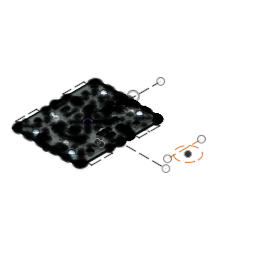
麦轮小车底盘上板-可编辑 (Autodesk Fusion 360 design; units mm, degrees)
Autodesk Fusion 360 part; units mm, degrees
(part 1 of 2)
sketch "草图1" plane through (0, 0, 0) normal (0, 0, 1) x (1, 0, 0)
  circle A0 centre (53, 101) radius 2.1
  line L0 (45.5, 106) -> (86.5, 106) construction
  line L1 (86.5, 106) -> (86.5, 66) construction
  line L2 (86.5, 66) -> (45.5, 66) construction
  line L3 (45.5, 66) -> (45.5, 106) construction
  circle A1 centre (78, 101) radius 2.1
  circle A2 centre (53, 71) radius 2.1
  circle A3 centre (78, 71) radius 2.1
  line L4 (83.5, 106) -> (83.5, 66) construction
  circle A4 centre (277.8426, 86) radius 37.5 construction
  line L5 (86.5, 86) -> (45.5, 86) construction
  line L6 (255.8426, 157.1035) -> (255.8426, 33.728) construction
  line L7 (0, 0) -> (284.0564, 0) construction
  line L8 (0, 0) -> (0, 265.0446) construction
  line L9 (122, 150) -> (-122, 150) construction
  line L10 (-122, 150) -> (-122, -150)
  line L11 (-122, -150) -> (122, -150) construction
  line L12 (122, -150) -> (122, 150)
  line L13 (122, 150) -> (-122, -150) construction
  line L14 (-122, 150) -> (122, -150) construction
  line L15 (13.5, 100) -> (45.5, 100) construction
  line L16 (45.5, 100) -> (45.5, 72) construction
  line L17 (45.5, 72) -> (13.5, 72) construction
  line L18 (13.5, 72) -> (13.5, 100) construction
  line L19 (86.5, 100) -> (106, 100) construction
  line L20 (106, 100) -> (106, 72) construction
  line L21 (106, 72) -> (86.5, 72) construction
  line L22 (86.5, 72) -> (86.5, 100) construction
  line L23 (106, 123.5) -> (138, 123.5) construction
  line L24 (138, 123.5) -> (138, 48.5) construction
  line L25 (138, 48.5) -> (106, 48.5) construction
  line L26 (106, 48.5) -> (106, 123.5) construction
  line L27 (86.5, 86) -> (138, 86) construction
  circle A5 centre (40.5, 61) radius 5 construction
  line L28 (-106, 123.5) -> (-138, 123.5) construction
  line L29 (-106, 48.5) -> (-106, 123.5) construction
  line L30 (-138, 48.5) -> (-106, 48.5) construction
  line L31 (-138, 123.5) -> (-138, 48.5) construction
  line L32 (-138, -123.5) -> (-138, -48.5) construction
  line L33 (-106, -123.5) -> (-138, -123.5) construction
  line L34 (-106, -48.5) -> (-106, -123.5) construction
  line L35 (-138, -48.5) -> (-106, -48.5) construction
  line L36 (106, -48.5) -> (106, -123.5) construction
  line L37 (106, -123.5) -> (138, -123.5) construction
  line L38 (138, -123.5) -> (138, -48.5) construction
  line L39 (138, -48.5) -> (106, -48.5) construction
  line L40 (117, 126.5) -> (99, 126.5) construction
  line L41 (96, 123.5) -> (96, 86) construction
  arc A6 (99, 126.5) -> (96, 123.5) centre (99, 123.5) ccw construction
  line L42 (96, 48.5) -> (96, 86) construction
  arc A7 (96, 48.5) -> (99, 45.5) centre (99, 48.5) ccw construction
  line L43 (117, 45.5) -> (99, 45.5) construction
  line L44 (122, 131.5) -> (122, 140)
  line L45 (112, 150) -> (0, 150)
  line L46 (122, 40.5) -> (122, 0)
  arc A8 (117, 126.5) -> (122, 131.5) centre (117, 131.5) ccw construction
  arc A9 (122, 40.5) -> (117, 45.5) centre (117, 40.5) ccw construction
  arc A10 (122, 140) -> (112, 150) centre (112, 140) ccw
  line L47 (-117, 45.5) -> (-99, 45.5) construction
  arc A11 (-99, 45.5) -> (-96, 48.5) centre (-99, 48.5) ccw construction
  line L48 (-122, 40.5) -> (-122, 0)
  arc A12 (-117, 45.5) -> (-122, 40.5) centre (-117, 40.5) ccw construction
  line L49 (-96, 48.5) -> (-96, 86) construction
  line L50 (-96, 123.5) -> (-96, 86) construction
  arc A13 (-96, 123.5) -> (-99, 126.5) centre (-99, 123.5) ccw construction
  line L51 (-117, 126.5) -> (-99, 126.5) construction
  arc A14 (-122, 131.5) -> (-117, 126.5) centre (-117, 131.5) ccw construction
  line L52 (-122, 131.5) -> (-122, 140)
  arc A15 (-112, 150) -> (-122, 140) centre (-112, 140) ccw
  line L53 (-112, 150) -> (0, 150)
  line L54 (-96, -123.5) -> (-96, -86) construction
  line L55 (-96, -48.5) -> (-96, -86) construction
  line L56 (-117, -45.5) -> (-99, -45.5) construction
  arc A16 (-96, -48.5) -> (-99, -45.5) centre (-99, -48.5) ccw construction
  arc A17 (-122, -40.5) -> (-117, -45.5) centre (-117, -40.5) ccw construction
  line L57 (-122, -40.5) -> (-122, 0)
  arc A18 (-99, -126.5) -> (-96, -123.5) centre (-99, -123.5) ccw construction
  line L58 (-117, -126.5) -> (-99, -126.5) construction
  arc A19 (-117, -126.5) -> (-122, -131.5) centre (-117, -131.5) ccw construction
  line L59 (-122, -131.5) -> (-122, -140)
  arc A20 (-122, -140) -> (-112, -150) centre (-112, -140) ccw
  line L60 (-112, -150) -> (0, -150)
  line L61 (112, -150) -> (0, -150)
  arc A21 (112, -150) -> (122, -140) centre (112, -140) ccw
  line L62 (122, -131.5) -> (122, -140)
  arc A22 (122, -131.5) -> (117, -126.5) centre (117, -131.5) ccw construction
  line L63 (117, -126.5) -> (99, -126.5) construction
  arc A23 (96, -123.5) -> (99, -126.5) centre (99, -123.5) ccw construction
  line L64 (96, -123.5) -> (96, -86) construction
  line L65 (96, -48.5) -> (96, -86) construction
  arc A24 (99, -45.5) -> (96, -48.5) centre (99, -48.5) ccw construction
  line L66 (117, -45.5) -> (99, -45.5) construction
  arc A25 (117, -45.5) -> (122, -40.5) centre (117, -40.5) ccw construction
  line L67 (122, -40.5) -> (122, 0)
  circle A26 centre (-40.5, 61) radius 5 construction
  circle A27 centre (-78, 71) radius 2.1
  circle A28 centre (-53, 71) radius 2.1
  circle A29 centre (-53, 101) radius 2.1
  circle A30 centre (-78, 101) radius 2.1
  circle A31 centre (40.5, -61) radius 5
  circle A32 centre (-40.5, -61) radius 5
  line L68 (-99, 45.5) -> (99, 45.5) construction
  line L69 (-96, 48.5) -> (-96, 45.5) construction
  line L70 (96, 48.5) -> (96, 45.5) construction
  line L71 (-93, 48.5) -> (93, 48.5) construction
  line L72 (-96, 86) -> (-96, 51.5) construction
  line L73 (96, 86) -> (96, 51.5) construction
  arc A33 (93, 48.5) -> (96, 51.5) centre (93, 51.5) ccw construction
  arc A34 (-96, 51.5) -> (-93, 48.5) centre (-93, 51.5) ccw construction
  line L74 (8, 91) -> (-8, 91) construction
  arc A35 (-8, 91) -> (-8, 81) centre (-8, 86) ccw construction
  line L75 (-8, 81) -> (8, 81) construction
  arc A36 (8, 81) -> (8, 91) centre (8, 86) ccw construction
  line L76 (8, 86) -> (-8, 86) construction
  line L77 (-8, -81) -> (8, -81)
  arc A37 (-8, -81) -> (-8, -91) centre (-8, -86) ccw
  line L78 (8, -91) -> (-8, -91)
  arc A38 (8, -91) -> (8, -81) centre (8, -86) ccw
  circle A39 centre (-78, -71) radius 2.1
  circle A40 centre (-78, -101) radius 2.1
  circle A41 centre (-53, -101) radius 2.1
  circle A42 centre (-53, -71) radius 2.1
  circle A43 centre (53, -101) radius 2.1
  circle A44 centre (78, -101) radius 2.1
  circle A45 centre (78, -71) radius 2.1
  circle A46 centre (53, -71) radius 2.1
  circle A47 centre (-112, 140) radius 2.1
  circle A48 centre (112, 140) radius 2.1
  circle A49 centre (-112, -140) radius 2.1
  circle A50 centre (112, -140) radius 2.1
  line L79 (92, 53) -> (87, 53) construction
  arc A51 (87, 53) -> (87, 50) centre (87, 51.5) ccw construction
  line L80 (87, 50) -> (92, 50) construction
  arc A52 (92, 50) -> (92, 53) centre (92, 51.5) ccw construction
  line L81 (92, 51.5) -> (87, 51.5) construction
  line L82 (92, 44) -> (87, 44) construction
  arc A53 (87, 44) -> (87, 41) centre (87, 42.5) ccw construction
  line L83 (87, 41) -> (92, 41) construction
  arc A54 (92, 41) -> (92, 44) centre (92, 42.5) ccw construction
  line L84 (92, 42.5) -> (87, 42.5) construction
  line L85 (-87, 50) -> (-92, 50) construction
  arc A55 (-87, 50) -> (-87, 53) centre (-87, 51.5) ccw construction
  line L86 (-92, 53) -> (-87, 53) construction
  arc A56 (-92, 53) -> (-92, 50) centre (-92, 51.5) ccw construction
  line L87 (-92, 44) -> (-87, 44) construction
  arc A57 (-87, 41) -> (-87, 44) centre (-87, 42.5) ccw construction
  line L88 (-87, 41) -> (-92, 41) construction
  arc A58 (-92, 44) -> (-92, 41) centre (-92, 42.5) ccw construction
  circle A59 centre (20.5, 39.5) radius 2.75 construction
  circle A60 centre (16, 54) radius 2.9 construction
  circle A61 centre (-16, 54) radius 2.9 construction
  circle A62 centre (-20.5, 39.5) radius 2.75 construction
  circle A63 centre (15.25, 15.25) radius 1.55
  circle A64 centre (22.5, 22.5) radius 1.55
  line L89 (0, 0) -> (46.5904, 46.5904) construction
  line L90 (0, 0) -> (50.6063, 0) construction
  circle A65 centre (-15.25, 15.25) radius 1.55
  circle A66 centre (-22.5, 22.5) radius 1.55
  circle A67 centre (22.5, -22.5) radius 1.55
  circle A68 centre (15.25, -15.25) radius 1.55
  circle A69 centre (-15.25, -15.25) radius 1.55
  circle A70 centre (-22.5, -22.5) radius 1.55
  circle A71 centre (0, 0) radius 5
  line L91 (116.45, 32.5) -> (116.45, 7.5)
  arc A72 (116.45, 7.5) -> (119.55, 7.5) centre (118, 7.5) ccw
  line L92 (119.55, 7.5) -> (119.55, 32.5)
  arc A73 (119.55, 32.5) -> (116.45, 32.5) centre (118, 32.5) ccw
  line L93 (118, 32.5) -> (118, 7.5) construction
  circle A74 centre (118, 0) radius 1.6
  circle A75 centre (118, 40) radius 1.6
  circle A76 centre (118, -40) radius 1.6
  line L94 (116.45, -32.5) -> (116.45, -7.5)
  arc A77 (116.45, -32.5) -> (119.55, -32.5) centre (118, -32.5) ccw
  line L95 (119.55, -7.5) -> (119.55, -32.5)
  arc A78 (119.55, -7.5) -> (116.45, -7.5) centre (118, -7.5) ccw
  circle A79 centre (-118, -40) radius 1.6
  arc A80 (-119.55, -32.5) -> (-116.45, -32.5) centre (-118, -32.5) ccw
  line L96 (-119.55, -7.5) -> (-119.55, -32.5)
  line L97 (-116.45, -32.5) -> (-116.45, -7.5)
  arc A81 (-116.45, -7.5) -> (-119.55, -7.5) centre (-118, -7.5) ccw
  circle A82 centre (-118, 0) radius 1.6
  arc A83 (-119.55, 7.5) -> (-116.45, 7.5) centre (-118, 7.5) ccw
  line L98 (-119.55, 7.5) -> (-119.55, 32.5)
  line L99 (-116.45, 32.5) -> (-116.45, 7.5)
  arc A84 (-116.45, 32.5) -> (-119.55, 32.5) centre (-118, 32.5) ccw
  circle A85 centre (-118, 40) radius 1.6
  line L100 (116.45, 141.5) -> (116.45, 131.5)
  arc A86 (116.45, 131.5) -> (119.55, 131.5) centre (118, 131.5) ccw
  line L101 (119.55, 131.5) -> (119.55, 141.5)
  arc A87 (119.55, 141.5) -> (116.45, 141.5) centre (118, 141.5) ccw
  line L102 (118, 141.5) -> (118, 131.5) construction
  line L103 (-119.55, 131.5) -> (-119.55, 141.5)
  line L104 (-116.45, 141.5) -> (-116.45, 131.5)
  arc A88 (-116.45, 141.5) -> (-119.55, 141.5) centre (-118, 141.5) ccw
  arc A89 (-119.55, 131.5) -> (-116.45, 131.5) centre (-118, 131.5) ccw
  line L105 (-15, 144.45) -> (15, 144.45)
  arc A90 (15, 144.45) -> (15, 147.55) centre (15, 146) ccw
  line L106 (15, 147.55) -> (-15, 147.55)
  arc A91 (-15, 147.55) -> (-15, 144.45) centre (-15, 146) ccw
  line L107 (-15, 146) -> (15, 146) construction
  circle A92 centre (22.5, 146) radius 1.6
  line L108 (30, 144.45) -> (60, 144.45)
  arc A93 (60, 144.45) -> (60, 147.55) centre (60, 146) ccw
  line L109 (60, 147.55) -> (30, 147.55)
  arc A94 (30, 147.55) -> (30, 144.45) centre (30, 146) ccw
  line L110 (30, 146) -> (60, 146) construction
  circle A95 centre (67.5, 146) radius 1.6
  line L111 (75, 144.45) -> (105, 144.45)
  arc A96 (105, 144.45) -> (105, 147.55) centre (105, 146) ccw
  line L112 (105, 147.55) -> (75, 147.55)
  arc A97 (75, 147.55) -> (75, 144.45) centre (75, 146) ccw
  line L113 (75, 146) -> (105, 146) construction
  circle A98 centre (112.5, 146) radius 1.6
  arc A99 (-30, 144.45) -> (-30, 147.55) centre (-30, 146) ccw
  line L114 (-60, 147.55) -> (-30, 147.55)
  arc A100 (-60, 147.55) -> (-60, 144.45) centre (-60, 146) ccw
  line L115 (-30, 144.45) -> (-60, 144.45)
  circle A101 centre (-67.5, 146) radius 1.6
  circle A102 centre (-22.5, 146) radius 1.6
  arc A103 (-75, 144.45) -> (-75, 147.55) centre (-75, 146) ccw
  line L116 (-105, 147.55) -> (-75, 147.55)
  line L117 (-75, 144.45) -> (-105, 144.45)
  arc A104 (-105, 147.55) -> (-105, 144.45) centre (-105, 146) ccw
  circle A105 centre (-112.5, 146) radius 1.6
  circle A106 centre (0, 135) radius 5
  circle A107 centre (40.5, 33) radius 5 construction
  circle A108 centre (45.5, 52.5) radius 1.5 construction
  line L118 (40.5, 61) -> (40.5, 33) construction
  circle A109 centre (35.5, 52.5) radius 1.5 construction
  circle A110 centre (35.5, 41.5) radius 1.5 construction
  circle A111 centre (45.5, 41.5) radius 1.5 construction
  circle A112 centre (-35.5, 52.5) radius 1.5 construction
  circle A113 centre (-45.5, 52.5) radius 1.5 construction
  circle A114 centre (-35.5, 41.5) radius 1.5 construction
  circle A115 centre (-45.5, 41.5) radius 1.5 construction
  circle A116 centre (-40.5, 33) radius 5 construction
  circle A117 centre (35.5, -52.5) radius 1.5
  circle A118 centre (45.5, -52.5) radius 1.5
  circle A119 centre (-35.5, -52.5) radius 1.5
  circle A120 centre (-45.5, -52.5) radius 1.5
  circle A121 centre (6, 76.5) radius 1.5
  circle A122 centre (-6, 76.5) radius 1.5
  circle A123 centre (0, 115) radius 25.5 construction
  circle A124 centre (0, 115) radius 19.8 construction
  line L119 (0, 115) -> (20.8597, 135.8596) construction
  line L120 (0, 115) -> (15.4307, 115) construction
  circle A125 centre (14.0007, 129.0007) radius 1.3
  circle A126 centre (-14.0007, 100.9993) radius 1.3
  circle A127 centre (0, 115) radius 29.5 construction
  circle A128 centre (20.8597, 135.8596) radius 1.6
  circle A129 centre (-20.8596, 135.8597) radius 1.6
  circle A130 centre (-20.8596, 94.1403) radius 1.6
  circle A131 centre (20.8597, 94.1403) radius 1.6
  circle A132 centre (-14.0007, 129.0007) radius 1.3
  circle A133 centre (14.0007, 100.9993) radius 1.3
  line L121 (-39.5, -73.5) -> (39.5, -73.5) construction
  line L122 (42.5, -76.5) -> (42.5, -126.5) construction
  line L123 (39.5, -129.5) -> (-39.5, -129.5) construction
  line L124 (-42.5, -126.5) -> (-42.5, -76.5) construction
  arc A134 (-39.5, -73.5) -> (-42.5, -76.5) centre (-39.5, -76.5) ccw construction
  arc A135 (42.5, -76.5) -> (39.5, -73.5) centre (39.5, -76.5) ccw construction
  arc A136 (39.5, -129.5) -> (42.5, -126.5) centre (39.5, -126.5) ccw construction
  arc A137 (-42.5, -126.5) -> (-39.5, -129.5) centre (-39.5, -126.5) ccw construction
  line L125 (-42.5, -101.5) -> (42.5, -101.5) construction
  circle A138 centre (-39, -77) radius 1.6
  circle A139 centre (-39, -126) radius 1.6
  circle A140 centre (19, -77) radius 1.6
  circle A141 centre (19, -126) radius 1.6
  line L126 (0, -73.5) -> (0, -129.5) construction
  circle A142 centre (-19, -77) radius 1.6
  circle A143 centre (39, -77) radius 1.6
  circle A144 centre (39, -126) radius 1.6
  circle A145 centre (-19, -126) radius 1.6
  line L127 (0, -101.5) -> (28.2843, -73.2157) construction
  line L128 (0, -101.5) -> (22.405, -101.5) construction
  circle A146 centre (24.5, -62.5) radius 1.6
  circle A147 centre (24.5, -82.5) radius 1.6
  circle A148 centre (24.5, -120.5) radius 1.6
  circle A149 centre (24.5, -140.5) radius 1.6
  circle A150 centre (-24.5, -140.5) radius 1.6
  circle A151 centre (-24.5, -120.5) radius 1.6
  circle A152 centre (-24.5, -82.5) radius 1.6
  circle A153 centre (-24.5, -62.5) radius 1.6
  circle A154 centre (-5, -61.5) radius 1.5
  circle A155 centre (5, -61.5) radius 1.5
  circle A156 centre (-5, -35) radius 1.5
  circle A157 centre (5, -35) radius 1.5
  circle A158 centre (5, 35) radius 1.5
  circle A159 centre (-5, 35) radius 1.5
  circle A160 centre (35, 5) radius 1.5
  circle A161 centre (35, -5) radius 1.5
  circle A162 centre (-35, 5) radius 1.5
  circle A163 centre (-35, -5) radius 1.5
  line L129 (-105, -147.55) -> (-75, -147.55)
  arc A164 (-105, -144.45) -> (-105, -147.55) centre (-105, -146) ccw
  circle A165 centre (-112.5, -146) radius 1.6
  line L130 (-75, -144.45) -> (-105, -144.45)
  arc A166 (-75, -147.55) -> (-75, -144.45) centre (-75, -146) ccw
  circle A167 centre (-67.5, -146) radius 1.6
  arc A168 (-60, -144.45) -> (-60, -147.55) centre (-60, -146) ccw
  line L131 (-60, -147.55) -> (-30, -147.55)
  line L132 (-30, -144.45) -> (-60, -144.45)
  arc A169 (-30, -147.55) -> (-30, -144.45) centre (-30, -146) ccw
  circle A170 centre (-22.5, -146) radius 1.6
  arc A171 (-15, -144.45) -> (-15, -147.55) centre (-15, -146) ccw
  line L133 (15, -147.55) -> (-15, -147.55)
  line L134 (-15, -144.45) -> (15, -144.45)
  arc A172 (15, -147.55) -> (15, -144.45) centre (15, -146) ccw
  circle A173 centre (22.5, -146) radius 1.6
  arc A174 (30, -144.45) -> (30, -147.55) centre (30, -146) ccw
  line L135 (60, -147.55) -> (30, -147.55)
  line L136 (30, -144.45) -> (60, -144.45)
  arc A175 (60, -147.55) -> (60, -144.45) centre (60, -146) ccw
  circle A176 centre (67.5, -146) radius 1.6
  arc A177 (75, -144.45) -> (75, -147.55) centre (75, -146) ccw
  line L137 (105, -147.55) -> (75, -147.55)
  line L138 (75, -144.45) -> (105, -144.45)
  arc A178 (105, -147.55) -> (105, -144.45) centre (105, -146) ccw
  circle A179 centre (112.5, -146) radius 1.6
  line L139 (116.45, -141.5) -> (116.45, -131.5)
  arc A180 (116.45, -141.5) -> (119.55, -141.5) centre (118, -141.5) ccw
  line L140 (119.55, -131.5) -> (119.55, -141.5)
  arc A181 (119.55, -131.5) -> (116.45, -131.5) centre (118, -131.5) ccw
  line L141 (-116.45, -141.5) -> (-116.45, -131.5)
  line L142 (-119.55, -131.5) -> (-119.55, -141.5)
  arc A182 (-119.55, -141.5) -> (-116.45, -141.5) centre (-118, -141.5) ccw
  arc A183 (-116.45, -131.5) -> (-119.55, -131.5) centre (-118, -131.5) ccw
  circle A184 centre (40, 140) radius 2.1
  circle A185 centre (-40, 140) radius 2.1
  circle A186 centre (-86, 58.5) radius 2.1
  circle A187 centre (86, 58.5) radius 2.1
  circle A188 centre (-112, 35.5) radius 2.1
  circle A189 centre (112, 35.5) radius 2.1
  circle A190 centre (112, -35.5) radius 2.1
  circle A191 centre (91, 86) radius 2.1
  circle A192 centre (-91, 86) radius 2.1
  circle A193 centre (91, -86) radius 2.1
  circle A194 centre (-91, -86) radius 2.1
  circle A195 centre (86, 113.5) radius 2.1
  circle A196 centre (-86, 113.5) radius 2.1
  circle A197 centre (86, -58.5) radius 2.1
  circle A198 centre (86, -113.5) radius 2.1
  circle A199 centre (-86, -113.5) radius 2.1
  circle A200 centre (-86, -58.5) radius 2.1
  circle A201 centre (30.5, 30.5) radius 2.1
  circle A202 centre (-30.5, 30.5) radius 2.1
  circle A203 centre (-30.5, -30.5) radius 2.1
  circle A204 centre (30.5, -30.5) radius 2.1
  circle A205 centre (-40, -140) radius 2.1
  circle A206 centre (40, -140) radius 2.1
  line L143 (62, 40) -> (102, 40) construction
  line L144 (102, 40) -> (102, -40) construction
  line L145 (102, -40) -> (62, -40) construction
  line L146 (62, -40) -> (62, 40) construction
  line L147 (58, 15) -> (58, -15)
  arc A207 (58, -15) -> (62, -15) centre (60, -15) ccw
  line L148 (62, -15) -> (62, 15)
  arc A208 (62, 15) -> (58, 15) centre (60, 15) ccw
  line L149 (60, 15) -> (60, -15) construction
  line L150 (82, 40) -> (82, -40) construction
  arc A209 (106, 15) -> (102, 15) centre (104, 15) ccw
  line L151 (106, 15) -> (106, -15)
  line L152 (102, -15) -> (102, 15)
  arc A210 (102, -15) -> (106, -15) centre (104, -15) ccw
  arc A211 (-106, -15) -> (-102, -15) centre (-104, -15) ccw
  line L153 (-106, 15) -> (-106, -15)
  arc A212 (-102, 15) -> (-106, 15) centre (-104, 15) ccw
  line L154 (-102, -15) -> (-102, 15)
  arc A213 (-58, 15) -> (-62, 15) centre (-60, 15) ccw
  line L155 (-58, 15) -> (-58, -15)
  arc A214 (-62, -15) -> (-58, -15) centre (-60, -15) ccw
  line L156 (-62, -15) -> (-62, 15)
  circle A215 centre (-112, -35.5) radius 2.1
  circle A216 centre (0, -47) radius 5 construction
  circle A217 centre (0, 115) radius 37.5 construction
  line L157 (0, 115) -> (16.1318, 76.0543) construction
  line L158 (0, 115) -> (42.1545, 115) construction
  circle A218 centre (9.7584, 91.4411) radius 1.6
  circle A219 centre (-9.7584, 91.4411) radius 1.6
  circle A220 centre (9.7584, 138.5589) radius 1.6
  circle A221 centre (-9.7584, 138.5589) radius 1.6
  line L159 (0, 115) -> (26.0167, 125.7765) construction
  line L160 (0, 115) -> (28.1603, 115) construction
  circle A222 centre (23.5589, 124.7584) radius 1.6
  circle A223 centre (23.5589, 105.2416) radius 1.6
  circle A224 centre (-23.5589, 124.7584) radius 1.6
  circle A225 centre (-23.5589, 105.2416) radius 1.6
  line L161 (-7.5, 61) -> (7.5, 61)
  arc A226 (7.5, 61) -> (7.5, 71) centre (7.5, 66) ccw
  line L162 (7.5, 71) -> (-7.5, 71)
  arc A227 (-7.5, 71) -> (-7.5, 61) centre (-7.5, 66) ccw
  line L163 (-7.5, 66) -> (7.5, 66) construction
  circle A228 centre (88.98, -110) radius 1.6
  circle A229 centre (-43.1, -110) radius 1.6
  circle A230 centre (-115.49, -110) radius 1.6
  circle A231 centre (88.98, 47.48) radius 1.6 construction
  circle A232 centre (-43.1, 47.48) radius 1.6
  circle A233 centre (111.84, 47.48) radius 1.6
  circle A234 centre (-115.49, 47.48) radius 1.6
  circle A235 centre (-43.1, 93.2) radius 1.6
  circle A236 centre (111.84, 93.2) radius 1.6
  circle A237 centre (-43.1, 113.52) radius 1.6
  line L164 (87, -7.5) -> (87, 7.5)
  arc A238 (87, 7.5) -> (77, 7.5) centre (82, 7.5) ccw
  line L165 (77, 7.5) -> (77, -7.5)
  arc A239 (77, -7.5) -> (87, -7.5) centre (82, -7.5) ccw
  line L166 (82, -7.5) -> (82, 7.5) construction
  arc A240 (-77, 7.5) -> (-87, 7.5) centre (-82, 7.5) ccw
  line L167 (-87, -7.5) -> (-87, 7.5)
  line L168 (-77, 7.5) -> (-77, -7.5)
  arc A241 (-87, -7.5) -> (-77, -7.5) centre (-82, -7.5) ccw
  circle A242 centre (37.78, -69) radius 1.6
  circle A243 centre (37.78, -121.07) radius 1.6
  circle A244 centre (-37.78, -121.07) radius 1.6
  circle A245 centre (-37.78, -69) radius 1.6
  line L169 (-7.5, -52) -> (7.5, -52)
  arc A246 (7.5, -52) -> (7.5, -42) centre (7.5, -47) ccw
  line L170 (7.5, -42) -> (-7.5, -42)
  arc A247 (-7.5, -42) -> (-7.5, -52) centre (-7.5, -47) ccw
  line L171 (-7.5, -47) -> (7.5, -47) construction
  line L172 (89.1958, -35) -> (74.1958, -35)
  arc A248 (74.1958, -35) -> (74.1958, -45) centre (74.1958, -40) ccw
  line L173 (74.1958, -45) -> (89.1958, -45)
  arc A249 (89.1958, -45) -> (89.1958, -35) centre (89.1958, -40) ccw
  line L174 (89.1958, -40) -> (74.1958, -40) construction
  line L175 (-74.1958, -45) -> (-89.1958, -45)
  arc A250 (-74.1958, -45) -> (-74.1958, -35) centre (-74.1958, -40) ccw
  line L176 (-89.1958, -35) -> (-74.1958, -35)
  arc A251 (-89.1958, -35) -> (-89.1958, -45) centre (-89.1958, -40) ccw
  line L177 (74.7, 48.34) -> (89.3, 48.34)
  line L178 (89.5, 48.14) -> (89.5, 40.2)
  line L179 (89.3, 40) -> (74.7, 40)
  line L180 (74.5, 40.2) -> (74.5, 48.14)
  arc A252 (74.7, 48.34) -> (74.5, 48.14) centre (74.7, 48.14) ccw
  arc A253 (74.5, 40.2) -> (74.7, 40) centre (74.7, 40.2) ccw
  arc A254 (89.5, 48.14) -> (89.3, 48.34) centre (89.3, 48.14) ccw
  arc A255 (89.3, 40) -> (89.5, 40.2) centre (89.3, 40.2) ccw
  circle A256 centre (71.75, 44.17) radius 1.3
  circle A257 centre (92.25, 44.17) radius 1.3
  line L181 (74.5, 44.17) -> (89.5, 44.17) construction
  circle A258 centre (-92.25, 44.17) radius 1.3
  line L182 (-89.5, 48.14) -> (-89.5, 40.2)
  line L183 (-74.5, 40.2) -> (-74.5, 48.14)
  line L184 (-74.7, 48.34) -> (-89.3, 48.34)
  arc A259 (-74.5, 48.14) -> (-74.7, 48.34) centre (-74.7, 48.14) ccw
  circle A260 centre (-71.75, 44.17) radius 1.3
  arc A261 (-74.7, 40) -> (-74.5, 40.2) centre (-74.7, 40.2) ccw
  line L185 (-89.3, 40) -> (-74.7, 40)
  arc A262 (-89.5, 40.2) -> (-89.3, 40) centre (-89.3, 40.2) ccw
  arc A263 (-89.3, 48.34) -> (-89.5, 48.14) centre (-89.3, 48.14) ccw
  circle A264 centre (65.0738, -123.4519) radius 11
  circle A265 centre (-65.0738, -123.4519) radius 11
  circle A266 centre (-65.0738, 123.4519) radius 11
  circle A267 centre (65.0738, 123.4519) radius 11
  point P0 (0, 86)
  point P1 (-42.5, -73.5)
  point P2 (42.5, -73.5)
  point P3 (-42.5, -129.5)
  point P4 (62, 0)
  point P5 (60, 0)
  point P6 (0, 66)
  point P7 (82, 0)
  point P8 (0, -47)
  point P9 (82, -40)
  point P10 (74.5, 48.34)
  point P11 (89.5, 48.34)
  point P12 (74.5, 40)
  dimension "d1" = 4.2
  dimension "d2" = 41
  dimension "d3" = 40
  dimension "d4" = 4.2
  dimension "d5" = 4.2
  dimension "d6" = 4.2
  dimension "d7" = 8.5
  dimension "d8" = 7.5
  dimension "d9" = 5
  dimension "d10" = 5
  dimension "d11" = 3
  dimension "d12" = 75
  dimension "d13" = 22
  dimension "d15" = 300
  dimension "d16" = 73
  dimension "d17" = 28
  dimension "d18" = 19.5
  dimension "d19" = 75
  dimension "d20" = 32
  dimension "d21" = 28
  dimension "d22" = 10
  dimension "d26" = 16
  dimension "d27" = 64
  dimension "d28" = 244
  dimension "d29" = 10
  dimension "d30" = 3
  dimension "d31" = 3
  dimension "d32" = 5
  dimension "d33" = 10
  dimension "d34" = 3
  dimension "d35" = 3
  dimension "d36" = 16
  dimension "d37" = 5
  dimension "d40" = 4.2
  dimension "d41" = 4.2
  dimension "d42" = 4.2
  dimension "d43" = 4.2
  dimension "d44" = 3
  dimension "d45" = 5
  dimension "d46" = 4
  dimension "d47" = 3
  dimension "d48" = 3
  dimension "d49" = 3
  dimension "d50" = 5.5
  dimension "d51" = 20.5
  dimension "d56" = 6
  dimension "d57" = 5.8
  dimension "d58" = 14.5
  dimension "d59" = 16
  dimension "d60" = 3.1
  dimension "d61" = 3.1
  dimension "d62" = 45
  dimension "d63" = 15.25
  dimension "d64" = 22.5
  dimension "d65" = 10
  dimension "d66" = 3.1
  dimension "d67" = 25
  dimension "d68" = 4
  dimension "d70" = 3.2
  dimension "d72" = 3.2
  dimension "d73" = 7.5
  dimension "d74" = 7.5
  dimension "d75" = 3.1
  dimension "d76" = 10
  dimension "d77" = 4
  dimension "d78" = 5
  dimension "d79" = 3.1
  dimension "d80" = 4
  dimension "d81" = 30
  dimension "d82" = 3.2
  dimension "d83" = 7.5
  dimension "d84" = 3.1
  dimension "d85" = 30
  dimension "d86" = 7.5
  dimension "d87" = 3.2
  dimension "d88" = 7.5
  dimension "d89" = 3.1
  dimension "d90" = 7.5
  dimension "d91" = 30
  dimension "d92" = 3.2
  dimension "d93" = 7.5
  dimension "d94" = 10
  dimension "d95" = 15
  dimension "d100" = 10
  dimension "d101" = 12.5
  dimension "d102" = 3
  dimension "d103" = 3
  dimension "d104" = 10
  dimension "d105" = 8.5
  dimension "d106" = 3
  dimension "d107" = 3
  dimension "d108" = 10
  dimension "d109" = 8.5
  dimension "d110" = 3
  dimension "d111" = 3
  dimension "d112" = 10
  dimension "d113" = 8.5
  dimension "d114" = 3
  dimension "d116" = 6
  dimension "d117" = 9.5
  dimension "d118" = 51
  dimension "d119" = 39.6
  dimension "d120" = 45
  dimension "d121" = 2.6
  dimension "d122" = 2.6
  dimension "d123" = 59
  dimension "d124" = 3.2
  dimension "d126" = 360
  dimension "d127" = 35
  dimension "d128" = 85
  dimension "d129" = 56
  dimension "d130" = 3
  dimension "d131" = 3.2
  dimension "d132" = 3.5
  dimension "d133" = 3.5
  dimension "d134" = 3.2
  dimension "d135" = 3.5
  dimension "d136" = 58
  dimension "d137" = 45
  dimension "d138" = 40
  dimension "d139" = 3
  dimension "d140" = 3
  dimension "d141" = 10
  dimension "d142" = 12
  dimension "d143" = 3
  dimension "d144" = 3
  dimension "d145" = 10
  dimension "d146" = 35
  dimension "d149" = 4.2
  dimension "d150" = 10
  dimension "d151" = 40
  dimension "d152" = 4.2
  dimension "d153" = 10
  dimension "d154" = 10
  dimension "d155" = 4.2
  dimension "d156" = 10
  dimension "d157" = 10
  dimension "d158" = 4.2
  dimension "d159" = 10
  dimension "d160" = 10
  dimension "d163" = 4.2
  dimension "d164" = 5
  dimension "d165" = 4.2
  dimension "d166" = 15
  dimension "d169" = 40
  dimension "d170" = 80
  dimension "d171" = 4
  dimension "d172" = 30
  dimension "d173" = 20
  dimension "d176" = 10
  dimension "d177" = 12
  dimension "d179" = 75
  dimension "d180" = 67.5
  dimension "d181" = 3.2
  dimension "d182" = 22.5
  dimension "d183" = 3.2
  dimension "d184" = 5
  dimension "d186" = 15
  dimension "d187" = 66
  dimension "d188" = 3.2
  dimension "d189" = 33.02
  dimension "d190" = 40
  dimension "d191" = 3.2
  dimension "d192" = 165.1
  dimension "d193" = 3.2
  dimension "d194" = 72.39
  dimension "d195" = 3.2
  dimension "d196" = 157.48
  dimension "d197" = 3.2
  dimension "d198" = 132.08
  dimension "d199" = 3.2
  dimension "d200" = 22.86
  dimension "d201" = 3.2
  dimension "d202" = 72.39
  dimension "d203" = 3.2
  dimension "d204" = 3.2
  dimension "d205" = 3.2
  dimension "d206" = 45.72
  dimension "d207" = 20.32
  dimension "d208" = 10
  dimension "d209" = 15
  dimension "d212" = 3.2
  dimension "d213" = 3.2
  dimension "d214" = 52.07
  dimension "d215" = 37.78
  dimension "d216" = 69
  dimension "d221" = 10
  dimension "d222" = 15
  dimension "d223" = 10
  dimension "d224" = 15
  dimension "d225" = 15
  dimension "d226" = 8.34
  dimension "d227" = 0.2
  dimension "d228" = 2.6
  dimension "d229" = 2.6
  dimension "d230" = 20.5
  dimension "d231" = 22
  constraint horizontal L0
  constraint vertical L1
  constraint horizontal L2
  constraint vertical L3
  constraint vertical A1.centre A3.centre
  constraint horizontal A2.centre A3.centre
  constraint vertical A0.centre A2.centre
  constraint horizontal A0.centre A1.centre
  constraint coincident L0 L4.start
  constraint coincident L2 L4.end
  constraint perpendicular L2 L4
  constraint coincident L1 L5.start
  constraint coincident L3 L5.end
  constraint perpendicular L3 L5
  constraint midpoint L3 L5.end
  constraint coincident A4.centre L5
  constraint vertical L6
  constraint coincident L7.start L8.start
  constraint horizontal L7
  constraint perpendicular L7 L8
  constraint horizontal L9
  constraint perpendicular L9 L10
  constraint parallel L9 L11
  constraint parallel L10 L12
  constraint coincident L13 L7.start
  constraint coincident L14 L7.start
  constraint horizontal L15
  constraint vertical L16
  constraint horizontal L17
  constraint vertical L18
  constraint coincident L3 L16.end
  constraint midpoint L5.end L16
  constraint horizontal L19
  constraint vertical L20
  constraint horizontal L21
  constraint vertical L22
  constraint coincident L1 L19.start
  constraint horizontal L23
  constraint vertical L24
  constraint horizontal L25
  constraint vertical L26
  constraint midpoint L5.start L22
  constraint coincident L24 L27.end
  constraint perpendicular L24 L27
  constraint collinear L20 L26
  constraint symmetric L23 L25 L27
  constraint tangent L2 A5
  constraint tangent L3 A5
  constraint symmetric L8 L23.start L28.start
  constraint symmetric L8 L23.end L28.end
  constraint symmetric L8 L24.end L30.start
  constraint symmetric L8 L25.end L29.start
  constraint symmetric L7 L23.start L36.end
  constraint symmetric L7 L23.end L37.end
  constraint symmetric L7 L24.end L38.end
  constraint symmetric L7 L25.end L36.start
  constraint symmetric L7 L28.start L33.start
  constraint symmetric L7 L28.end L32.start
  constraint symmetric L7 L29.start L34.start
  constraint symmetric L7 L30.start L32.end
  constraint perpendicular L12 L40
  constraint coincident L27 L41.end
  constraint perpendicular L27 L41
  constraint tangent L40 A6
  constraint tangent L41 A6
  constraint symmetric L27 L41.end L42.end
  constraint symmetric L27 L40.end A7.end
  constraint symmetric L27 L41.start L42.start
  constraint symmetric L27 A6 A7
  constraint midpoint L9 L45.end
  constraint midpoint L12 L46.end
  constraint tangent L40 A8
  constraint tangent L44 A8
  constraint tangent L43 A9
  constraint tangent L46 A9
  constraint equal A8 A9
  constraint vertical L44
  constraint vertical L46
  constraint horizontal L43
  constraint coincident L9.start L45
  constraint coincident L9.start L44
  constraint tangent L45 A10
  constraint tangent L44 A10
  constraint symmetric L8 L41.end L49.end
  constraint symmetric L8 L40.end A13.end
  constraint symmetric L8 L41.start L50.start
  constraint symmetric L8 A6 A13
  constraint symmetric L8 L42.start A11.end
  constraint symmetric L8 A7.end L47.end
  constraint symmetric L8 A7 A11
  constraint symmetric L8 L45.end L53.end
  constraint symmetric L8 L46.end L48.end
  constraint symmetric L8 L40.start L51.start
  constraint symmetric L8 L44.start A14.start
  constraint symmetric L8 A8 A14
  constraint symmetric L8 L43.start L47.start
  constraint symmetric L8 L46.start L48.start
  constraint symmetric L8 A9 A12
  constraint symmetric L8 L45.start A15.start
  constraint symmetric L8 L44.end L52.end
  constraint symmetric L8 A10 A15
  constraint symmetric L7 L41.end L64.end
  constraint symmetric L7 L40.end L63.end
  constraint symmetric L7 L41.start A23.start
  constraint symmetric L7 A6 A23
  constraint symmetric L7 L42.start L65.start
  constraint symmetric L7 A7.end A24.start
  constraint symmetric L7 A7 A24
  constraint symmetric L7 L45.end L60.end
  constraint symmetric L7 L46.end L67.end
  constraint symmetric L7 L40.start A22.end
  constraint symmetric L7 L44.start L62.start
  constraint symmetric L7 A8 A22
  constraint symmetric L7 L43.start L66.start
  constraint symmetric L7 L46.start A25.end
  constraint symmetric L7 A9 A25
  constraint symmetric L7 L45.start L61.start
  constraint symmetric L7 L44.end A21.end
  constraint symmetric L7 A10 A21
  constraint symmetric L7 L47.start L56.start
  constraint symmetric L7 L47.end L56.end
  constraint symmetric L7 A11.end L55.start
  constraint symmetric L7 A11 A16
  constraint symmetric L7 L48.start A17.start
  constraint symmetric L7 L48.end L57.end
  constraint symmetric L7 A12 A17
  constraint symmetric L7 L49.end L54.end
  constraint symmetric L7 L50.start L54.start
  constraint symmetric L7 A13.end A18.start
  constraint symmetric L7 A13 A18
  constraint symmetric L7 L51.start L58.start
  constraint symmetric L7 A14.start A19.end
  constraint symmetric L7 A14 A19
  constraint symmetric L7 L52.end L59.end
  constraint symmetric L7 A15.start A20.end
  constraint symmetric L7 A15 A20
  constraint symmetric A0 L8 A29
  constraint symmetric A1 L8 A30
  constraint symmetric A2 L8 A28
  constraint symmetric A3 L8 A27
  constraint symmetric L8 A5 A26
  constraint symmetric L7 A5 A31
  constraint symmetric L7 A26 A32
  constraint coincident L68 L69.end
  constraint tangent A11 L69
  constraint coincident L68 L70.end
  constraint tangent A7 L70
  constraint horizontal L71
  constraint tangent A7 L73
  constraint tangent L73 A33
  constraint tangent L71 A33
  constraint tangent L71 A34
  constraint tangent L72 A34
  constraint equal A33 A34
  constraint tangent L74 A35
  constraint tangent A35 L75
  constraint parallel L74 L75
  constraint tangent L75 A36
  constraint tangent L74 A36
  constraint perpendicular L8 L76
  constraint coincident L8 P0
  constraint midpoint L76 P0
  constraint collinear L5 L76
  constraint symmetric L7 L74.start L78.start
  constraint symmetric L7 L74.end A37.end
  constraint symmetric L7 A35.end L77.start
  constraint symmetric L7 L75.end L77.end
  constraint symmetric L7 A35 A37
  constraint symmetric L7 A36 A38
  constraint symmetric A0 L7 A43
  constraint symmetric A1 L7 A44
  constraint symmetric A2 L7 A46
  constraint symmetric A3 L7 A45
  constraint symmetric L7 A27 A39
  constraint symmetric L7 A28 A42
  constraint symmetric L7 A29 A41
  constraint symmetric L7 A30 A40
  constraint concentric A15 A47
  constraint concentric A10 A48
  constraint concentric A20 A49
  constraint concentric A21 A50
  constraint tangent L79 A51
  constraint tangent A51 L80
  constraint parallel L79 L80
  constraint tangent L80 A52
  constraint tangent L79 A52
  constraint parallel L71 L81
  constraint tangent L82 A53
  constraint tangent A53 L83
  constraint parallel L82 L83
  constraint tangent L83 A54
  constraint tangent L82 A54
  constraint parallel L68 L84
  constraint vertical A52.centre A54.centre
  constraint vertical A51.centre A53.centre
  constraint symmetric L8 L79.start L86.start
  constraint symmetric L8 L79.end A55.end
  constraint symmetric L8 A51.end L85.start
  constraint symmetric L8 L80.end L85.end
  constraint symmetric L8 A51 A55
  constraint symmetric L8 A52 A56
  constraint symmetric L8 L82.start L87.start
  constraint symmetric L8 L82.end L87.end
  constraint symmetric L8 A53.end A57.start
  constraint symmetric L8 L83.end L88.end
  constraint symmetric L8 A53 A57
  constraint symmetric L8 A54 A58
  constraint vertical L72
  constraint symmetric L8 A59 A62
  constraint symmetric L8 A60 A61
  constraint horizontal L90
  constraint coincident A64.centre L89
  constraint coincident A63.centre L89
  constraint symmetric L8 A63 A65
  constraint symmetric L8 A64 A66
  constraint symmetric L7 A63 A68
  constraint symmetric L7 A64 A67
  constraint symmetric L7 A65 A69
  constraint symmetric L7 A66 A70
  constraint tangent L91 A72
  constraint tangent A72 L92
  constraint parallel L91 L92
  constraint tangent L92 A73
  constraint tangent L91 A73
  constraint perpendicular L68 L93
  constraint coincident L7 A74.centre
  constraint symmetric L7 L91.start L94.start
  constraint symmetric L7 L91.end L94.end
  constraint symmetric L7 A72.end L95.start
  constraint symmetric L7 L92.end A77.end
  constraint symmetric L7 A72 A78
  constraint symmetric L7 A73 A77
  constraint symmetric L7 A75 A76
  constraint symmetric L8 L91.start L99.start
  constraint symmetric L8 L91.end A83.end
  constraint symmetric L8 A72.end A83.start
  constraint symmetric L8 L92.end L98.end
  constraint symmetric L8 A72 A83
  constraint symmetric L8 A73 A84
  constraint symmetric L8 A74 A82
  constraint symmetric L8 A75 A85
  constraint symmetric L8 A76 A79
  constraint symmetric L8 L94.start A80.end
  constraint symmetric L8 L94.end L97.end
  constraint symmetric L8 A77.end A80.start
  constraint symmetric L8 A77 A80
  constraint symmetric L8 L95.start L96.start
  constraint symmetric L8 A78 A81
  constraint coincident L93 A74.centre
  constraint coincident L93 A75.centre
  constraint tangent L100 A86
  constraint tangent A86 L101
  constraint parallel L100 L101
  constraint tangent L101 A87
  constraint tangent L100 A87
  constraint vertical L102
  constraint symmetric L8 L100.start L104.start
  constraint symmetric L8 L100.end L104.end
  constraint symmetric L8 A86.end L103.start
  constraint symmetric L8 L101.end L103.end
  constraint symmetric L8 A86 A89
  constraint symmetric L8 A87 A88
  constraint tangent L105 A90
  constraint tangent A90 L106
  constraint parallel L105 L106
  constraint tangent L106 A91
  constraint tangent L105 A91
  constraint parallel L53 L107
  constraint symmetric L8 A91.centre A90.centre
  constraint coincident L107 A92.centre
  constraint tangent L108 A93
  constraint tangent A93 L109
  constraint parallel L108 L109
  constraint tangent L109 A94
  constraint tangent L108 A94
  constraint horizontal L110
  constraint collinear L107 L110
  constraint coincident L110 A95.centre
  constraint tangent L111 A96
  constraint tangent A96 L112
  constraint parallel L111 L112
  constraint tangent L112 A97
  constraint tangent L111 A97
  constraint parallel L45 L113
  constraint coincident L113 A98.centre
  constraint collinear L107 L113
  constraint symmetric L8 A92 A102
  constraint symmetric L8 L108.start A99.start
  constraint symmetric L8 L108.end A100.end
  constraint symmetric L8 A93.end L114.start
  constraint symmetric L8 L109.end A99.end
  constraint symmetric L8 A93 A100
  constraint symmetric L8 A94 A99
  constraint symmetric L8 A95 A101
  constraint symmetric L8 L111.start A103.start
  constraint symmetric L8 L111.end L117.end
  constraint symmetric L8 A96.end L116.start
  constraint symmetric L8 L112.end A103.end
  constraint symmetric L8 A96 A104
  constraint symmetric L8 A97 A103
  constraint symmetric L8 A98 A105
  constraint coincident L8 A106.centre
  constraint vertical A5.centre A107.centre
  constraint coincident A5.centre L118.start
  constraint coincident A107.centre L118.end
  constraint horizontal A108.centre A109.centre
  constraint symmetric A108 L118 A109
  constraint horizontal A110.centre A111.centre
  constraint symmetric L118 A110 A111
  constraint symmetric L8 A107 A116
  constraint symmetric L8 A108 A113
  constraint symmetric L8 A109 A112
  constraint symmetric L8 A110 A114
  constraint symmetric L8 A111 A115
  constraint horizontal A118.centre A117.centre
  constraint symmetric L118 A117 A118
  constraint symmetric L8 A117 A119
  constraint symmetric L8 A118 A120
  constraint symmetric L8 A121 A122
  constraint coincident L8 A123.centre
  constraint concentric A123 A124
  constraint horizontal L120
  constraint coincident A123.centre A124.centre
  constraint coincident A124 A125.centre
  constraint coincident L119 A125.centre
  constraint coincident A124 A126.centre
  constraint coincident L119 A126.centre
  constraint concentric A124 A127
  constraint coincident L119.end A127
  constraint coincident L119.end A128.centre
  constraint symmetric L8 A125 A132
  constraint symmetric L8 A126 A133
  constraint horizontal L121
  constraint vertical L122
  constraint horizontal L123
  constraint vertical L124
  constraint coincident P1 L121
  constraint coincident P1 L124
  constraint tangent L121 A134
  constraint tangent L124 A134
  constraint coincident P2 L121
  constraint coincident P2 L122
  constraint tangent L121 A135
  constraint tangent L122 A135
  constraint equal A134 A135
  constraint tangent L122 A136
  constraint tangent L123 A136
  constraint equal A134 A136
  constraint coincident P3 L123
  constraint coincident P3 L124
  constraint tangent L123 A137
  constraint tangent L124 A137
  constraint equal A134 A137
  constraint coincident L124 L125.start
  constraint coincident L122 L125.end
  constraint perpendicular L122 L125
  constraint midpoint L124 L125.start
  constraint symmetric L125 A138 A139
  constraint symmetric L125 A140 A141
  constraint midpoint L121 L126.start
  constraint midpoint L123 L126.end
  constraint symmetric A138 L126 A143
  constraint symmetric A139 L126 A144
  constraint symmetric A140 L126 A142
  constraint symmetric A141 L126 A145
  constraint horizontal L128
  constraint midpoint L125 L127.start
  constraint symmetric A138 L127 A149
  constraint symmetric A139 L127 A150
  constraint symmetric A140 L127 A147
  constraint symmetric A141 L127 A152
  constraint symmetric A142 L127 A148
  constraint symmetric A143 L127 A146
  constraint symmetric A144 L127 A153
  constraint symmetric A145 L127 A151
  constraint collinear L8 L126
  constraint coincident A31.centre L127
  constraint symmetric L8 A154 A155
  constraint symmetric L8 A156 A157
  constraint symmetric L90 A156 A159
  constraint symmetric L90 A157 A158
  constraint symmetric L89 A158 A160
  constraint symmetric L89 A159 A161
  constraint symmetric L89 A156 A163
  constraint symmetric L89 A157 A162
  constraint symmetric L7 L100.start L139.start
  constraint symmetric L7 L100.end L139.end
  constraint symmetric L7 A86.end L140.start
  constraint symmetric L7 L101.end A180.end
  constraint symmetric L7 A86 A181
  constraint symmetric L7 A87 A180
  constraint symmetric L7 L103.start L142.start
  constraint symmetric L7 L103.end L142.end
  constraint symmetric L7 L104.start L141.start
  constraint symmetric L7 L104.end L141.end
  constraint symmetric L7 A88 A182
  constraint symmetric L7 A89 A183
  constraint symmetric L7 L105.start A171.start
  constraint symmetric L7 L105.end L134.end
  constraint symmetric L7 A90.end L133.start
  constraint symmetric L7 L106.end A171.end
  constraint symmetric L7 A90 A172
  constraint symmetric L7 A91 A171
  constraint symmetric L7 A92 A173
  constraint symmetric L7 L108.start A174.start
  constraint symmetric L7 L108.end L136.end
  constraint symmetric L7 A93.end L135.start
  constraint symmetric L7 L109.end A174.end
  constraint symmetric L7 A93 A175
  constraint symmetric L7 A94 A174
  constraint symmetric L7 A95 A176
  constraint symmetric L7 L111.start A177.start
  constraint symmetric L7 L111.end L138.end
  constraint symmetric L7 A96.end L137.start
  constraint symmetric L7 L112.end A177.end
  constraint symmetric L7 A96 A178
  constraint symmetric L7 A97 A177
  constraint symmetric L7 A98 A179
  constraint symmetric L7 A99.end L131.end
  constraint symmetric L7 A99.start L132.start
  constraint symmetric L7 A99 A169
  constraint symmetric L7 L114.start A168.end
  constraint symmetric L7 A100.end A168.start
  constraint symmetric L7 A100 A168
  constraint symmetric L7 A101 A167
  constraint symmetric L7 A102 A170
  constraint symmetric L7 A103.end L129.end
  constraint symmetric L7 A103.start L130.start
  constraint symmetric L7 A103 A166
  constraint symmetric L7 L116.start L129.start
  constraint symmetric L7 L117.end A164.start
  constraint symmetric L7 A104 A164
  constraint symmetric L7 A105 A165
  constraint symmetric L8 A184 A185
  constraint symmetric L8 A186 A187
  constraint symmetric L8 A188 A189
  constraint coincident L27 A191.centre
  constraint symmetric L8 A191 A192
  constraint symmetric L7 A191 A193
  constraint symmetric L7 A192 A194
  constraint symmetric L27 A187 A195
  constraint symmetric L27 A186 A196
  constraint symmetric L7 A186 A200
  constraint symmetric L7 A187 A197
  constraint symmetric L7 A195 A198
  constraint symmetric L7 A196 A199
  constraint coincident L89 A201.centre
  constraint symmetric L8 A201 A202
  constraint symmetric L7 A201 A204
  constraint symmetric L7 A202 A203
  constraint symmetric L7 A184 A206
  constraint symmetric L7 A185 A205
  constraint horizontal L143
  constraint vertical L144
  constraint horizontal L145
  constraint vertical L146
  constraint midpoint L146 P4
  constraint coincident L7 P4
  constraint tangent L147 A207
  constraint tangent A207 L148
  constraint parallel L147 L148
  constraint tangent L148 A208
  constraint tangent L147 A208
  constraint perpendicular L7 L149
  constraint coincident L7 P5
  constraint midpoint L149 P5
  constraint collinear L146 L148
  constraint midpoint L143 L150.start
  constraint midpoint L145 P9
  constraint symmetric L147.start L150 A209.start
  constraint symmetric L147.end L150 L151.end
  constraint symmetric A207.end L150 L152.start
  constraint symmetric L148.end L150 A209.end
  constraint symmetric A207 L150 A210
  constraint symmetric A208 L150 A209
  constraint symmetric L8 L147.start A213.start
  constraint symmetric L8 L147.end L155.end
  constraint symmetric L8 A207.end A214.start
  constraint symmetric L8 L148.end A213.end
  constraint symmetric L8 A207 A214
  constraint symmetric L8 A208 A213
  constraint symmetric L8 A209.end A212.start
  constraint symmetric L8 A209.start L153.start
  constraint symmetric L8 A209 A212
  constraint symmetric L8 L151.end A211.start
  constraint symmetric L8 L152.start A211.end
  constraint symmetric L8 A210 A211
  constraint symmetric L8 A190 A215
  constraint coincident L8 P8
  constraint concentric A123 A217
  constraint horizontal L158
  constraint coincident L157 A218.centre
  constraint symmetric L8 A218 A219
  constraint symmetric L120 A218 A220
  constraint symmetric L120 A219 A221
  constraint coincident A123 A218.centre
  constraint horizontal L160
  constraint coincident L159 A222.centre
  constraint coincident A123 A222.centre
  constraint symmetric L160 A222 A223
  constraint symmetric L8 A222 A224
  constraint symmetric L8 A223 A225
  constraint tangent L161 A226
  constraint tangent A226 L162
  constraint parallel L161 L162
  constraint tangent L162 A227
  constraint tangent L161 A227
  constraint perpendicular L8 L163
  constraint coincident L8 P6
  constraint midpoint L163 P6
  constraint horizontal A228.centre A229.centre
  constraint horizontal A229.centre A230.centre
  constraint vertical A228.centre A231.centre
  constraint horizontal A231.centre A232.centre
  constraint horizontal A231.centre A233.centre
  constraint horizontal A232.centre A234.centre
  constraint vertical A232.centre A235.centre
  constraint vertical A232.centre A237.centre
  constraint vertical A233.centre A236.centre
  constraint horizontal A235.centre A236.centre
  constraint tangent L164 A238
  constraint tangent A238 L165
  constraint parallel L164 L165
  constraint tangent L165 A239
  constraint tangent L164 A239
  constraint coincident L150 A238.centre
  constraint midpoint L150 P7
  constraint midpoint L166 P7
  constraint symmetric L8 L164.start L167.start
  constraint symmetric L8 L164.end A240.end
  constraint symmetric L8 A238.end A240.start
  constraint symmetric L8 L165.end L168.end
  constraint symmetric L8 A238 A240
  constraint symmetric L8 A239 A241
  constraint vertical A242.centre A243.centre
  constraint symmetric L8 A242 A245
  constraint symmetric L8 A243 A244
  constraint tangent L169 A246
  constraint tangent A246 L170
  constraint parallel L169 L170
  constraint tangent L170 A247
  constraint tangent L169 A247
  constraint horizontal L171
  constraint coincident P8 A216.centre
  constraint midpoint L171 P8
  constraint tangent L172 A248
  constraint tangent A248 L173
  constraint parallel L172 L173
  constraint tangent L173 A249
  constraint tangent L172 A249
  constraint coincident L145 A248.centre
  constraint perpendicular L150 L174
  constraint coincident P9 L150.end
  constraint symmetric L8 L172.start L176.start
  constraint symmetric L8 L172.end A250.end
  constraint symmetric L8 A248.end L175.start
  constraint symmetric L8 L173.end L175.end
  constraint symmetric L8 A248 A250
  constraint symmetric L8 A249 A251
  constraint horizontal L177
  constraint vertical L178
  constraint horizontal L179
  constraint vertical L180
  constraint coincident P10 L177
  constraint coincident P10 L180
  constraint tangent L177 A252
  constraint tangent L180 A252
  constraint coincident P12 L179
  constraint coincident P12 L180
  constraint tangent L179 A253
  constraint tangent L180 A253
  constraint equal A252 A253
  constraint coincident P11 L177
  constraint coincident P11 L178
  constraint tangent L177 A254
  constraint tangent L178 A254
  constraint equal A252 A254
  constraint tangent L178 A255
  constraint tangent L179 A255
  constraint equal A252 A255
  constraint symmetric L150 L178 L180
  constraint collinear L143 L179
  constraint symmetric L150 A256 A257
  constraint midpoint L180 L181.start
  constraint midpoint L178 L181.end
  constraint coincident A256.centre L181
  constraint symmetric L8 L177.start L184.start
  constraint symmetric L8 L180.end L183.end